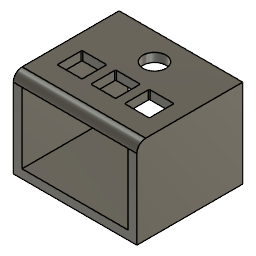
Lid (Autodesk Fusion 360 archive; units mm, degrees)
design "External1"
part number: 2026-05-08-13-42-59-027
Autodesk Fusion 360 part; units mm, degrees
other "DerivedContext1"
other "DerivedContext2"
sketch "sketch 238" plane through (0, 0, 0) normal (0, 1, 0) x (1, 0, 0)
  line L0 (35, -25) -> (-35, -25)
  line L1 (-35, -25) -> (-35, 25)
  line L2 (-35, 25) -> (35, 25)
  line L3 (35, 25) -> (35, -25)
  line L4 (35, -25) -> (-35, 25) construction
  line L5 (-35, -25) -> (35, 25) construction
extrude "Extrude1" add sketch "sketch 238" along normal blind 60
sketch "Sketch2" plane through (0, 0, 0) normal (0, -1, 0) x (1, 0, 0)
  line L0 (-35, -25) -> (35, -25)
  line L1 (35, -25) -> (35, 25)
  line L2 (35, 25) -> (-35, 25)
  line L3 (-35, 25) -> (-35, -25)
  line L4 (30, -20) -> (-30, -20)
  line L5 (-30, -20) -> (-30, 20)
  line L6 (-30, 20) -> (30, 20)
  line L7 (30, 20) -> (30, -20)
  line L8 (30, -20) -> (-30, 20) construction
  line L9 (-30, -20) -> (30, 20) construction
  dimension "d7" = 60
  dimension "d8" = 40
  constraint horizontal L4
  constraint perpendicular L4 L5
  constraint parallel L4 L6
  constraint parallel L5 L7
  constraint coincident L8 origin
  constraint coincident L9 origin
  measures "d7" distance of L5.end L6.end
  measures "d8" distance of L4.end L5.end
extrude "Extrude3" cut sketch "Sketch2" against normal blind 95 contours L4 L5 L6 L7
fillet "Fillet2" radius 5 1 edges at (0, 0, 25)
sketch "sketch 1124" plane through (28.575, 32.5, 25) normal (0, 0, 1) x (0, -1, 0)
  line L0 (3.025, -16.525) -> (16.025, -16.525)
  line L1 (2.525, -3.025) -> (2.525, -16.025)
  arc A0 (2.525, -16.025) -> (3.025, -16.525) centre (3.025, -16.025) ccw
  arc A1 (16.025, -16.525) -> (16.525, -16.025) centre (16.025, -16.025) ccw
  line L2 (3.025, -54.625) -> (16.025, -54.625)
  line L3 (0, 0) -> (19.05, 0)
  line L4 (16.525, -41.125) -> (16.525, -54.125)
  line L5 (2.525, -22.075) -> (2.525, -35.075)
  line L6 (0, -57.15) -> (0, 0)
  line L7 (16.525, -22.075) -> (16.525, -35.075)
  arc A2 (3.025, -2.525) -> (2.525, -3.025) centre (3.025, -3.025) ccw
  line L8 (3.025, -2.525) -> (16.025, -2.525)
  arc A3 (16.025, -54.625) -> (16.525, -54.125) centre (16.025, -54.125) ccw
  line L9 (3.025, -35.575) -> (16.025, -35.575)
  arc A4 (16.025, -35.575) -> (16.525, -35.075) centre (16.025, -35.075) ccw
  arc A5 (16.525, -41.125) -> (16.025, -40.625) centre (16.025, -41.125) ccw
  line L10 (19.05, -57.15) -> (19.05, 0)
  arc A6 (16.525, -3.025) -> (16.025, -2.525) centre (16.025, -3.025) ccw
  line L11 (16.525, -3.025) -> (16.525, -16.025)
  arc A7 (16.525, -22.075) -> (16.025, -21.575) centre (16.025, -22.075) ccw
  line L12 (0, -57.15) -> (19.05, -57.15)
  arc A8 (2.525, -35.075) -> (3.025, -35.575) centre (3.025, -35.075) ccw
  line L13 (3.025, -21.575) -> (16.025, -21.575)
  line L14 (2.525, -41.125) -> (2.525, -54.125)
  arc A9 (3.025, -40.625) -> (2.525, -41.125) centre (3.025, -41.125) ccw
  line L15 (3.025, -40.625) -> (16.025, -40.625)
  arc A10 (2.525, -54.125) -> (3.025, -54.625) centre (3.025, -54.125) ccw
  arc A11 (3.025, -21.575) -> (2.525, -22.075) centre (3.025, -22.075) ccw
extrude "Extrude4" cut sketch "sketch 1124" against normal blind 10 contours L0 L1 A0 A1 A2 L8 A6 L11 | L2 L4 A3 A5 L14 A9 L15 A10 | L5 L7 L9 A4 A7 A8 L13 A11
sketch "Sketch3" plane through (0, 0, 25) normal (0, 0, 1) x (-1, 0, 0)
  line L0 (25.55, -29.975) -> (12.55, -29.975)
  arc A0 (12.05, -29.475) -> (12.55, -29.975) centre (12.55, -29.475) ccw
  line L1 (12.05, -29.475) -> (12.05, -16.475)
  arc A1 (12.55, -15.975) -> (12.05, -16.475) centre (12.55, -16.475) ccw
  line L2 (12.55, -15.975) -> (25.55, -15.975)
  arc A2 (26.05, -16.475) -> (25.55, -15.975) centre (25.55, -16.475) ccw
  line L3 (26.05, -16.475) -> (26.05, -29.475)
  arc A3 (25.55, -29.975) -> (26.05, -29.475) centre (25.55, -29.475) ccw
  line L4 (-7, -29.475) -> (-7, -16.475)
  arc A4 (-6.5, -15.975) -> (-7, -16.475) centre (-6.5, -16.475) ccw
  line L5 (-6.5, -15.975) -> (6.5, -15.975)
  arc A5 (7, -16.475) -> (6.5, -15.975) centre (6.5, -16.475) ccw
  line L6 (7, -16.475) -> (7, -29.475)
  arc A6 (6.5, -29.975) -> (7, -29.475) centre (6.5, -29.475) ccw
  line L7 (6.5, -29.975) -> (-6.5, -29.975)
  arc A7 (-7, -29.475) -> (-6.5, -29.975) centre (-6.5, -29.475) ccw
  line L8 (-12.55, -29.975) -> (-25.55, -29.975)
  arc A8 (-26.05, -29.475) -> (-25.55, -29.975) centre (-25.55, -29.475) ccw
  line L9 (-26.05, -29.475) -> (-26.05, -16.475)
  arc A9 (-25.55, -15.975) -> (-26.05, -16.475) centre (-25.55, -16.475) ccw
  line L10 (-25.55, -15.975) -> (-12.55, -15.975)
  arc A10 (-12.05, -16.475) -> (-12.55, -15.975) centre (-12.55, -16.475) ccw
  line L11 (-12.05, -16.475) -> (-12.05, -29.475)
  arc A11 (-12.55, -29.975) -> (-12.05, -29.475) centre (-12.55, -29.475) ccw
  line L12 (35, -5) -> (-35, -5)
  line L13 (-35, -5) -> (-35, -60)
  line L14 (-35, -60) -> (35, -60)
  line L15 (35, -60) -> (35, -5)
  circle A12 centre (0, -45) radius 7.5
  dimension "d21" = 15
  measures "d21" diameter of A12
sketch "Sketch4" plane through (0, 0, 25) normal (0, 0, 1) x (-1, 0, 0)
  line L0 (25.55, -29.975) -> (12.55, -29.975)
  arc A0 (12.05, -29.475) -> (12.55, -29.975) centre (12.55, -29.475) ccw
  line L1 (12.05, -29.475) -> (12.05, -16.475)
  arc A1 (12.55, -15.975) -> (12.05, -16.475) centre (12.55, -16.475) ccw
  line L2 (12.55, -15.975) -> (25.55, -15.975)
  arc A2 (26.05, -16.475) -> (25.55, -15.975) centre (25.55, -16.475) ccw
  line L3 (26.05, -16.475) -> (26.05, -29.475)
  arc A3 (25.55, -29.975) -> (26.05, -29.475) centre (25.55, -29.475) ccw
  line L4 (-7, -29.475) -> (-7, -16.475)
  arc A4 (-6.5, -15.975) -> (-7, -16.475) centre (-6.5, -16.475) ccw
  line L5 (-6.5, -15.975) -> (6.5, -15.975)
  arc A5 (7, -16.475) -> (6.5, -15.975) centre (6.5, -16.475) ccw
  line L6 (7, -16.475) -> (7, -29.475)
  arc A6 (6.5, -29.975) -> (7, -29.475) centre (6.5, -29.475) ccw
  line L7 (6.5, -29.975) -> (-6.5, -29.975)
  arc A7 (-7, -29.475) -> (-6.5, -29.975) centre (-6.5, -29.475) ccw
  line L8 (-12.55, -29.975) -> (-25.55, -29.975)
  arc A8 (-26.05, -29.475) -> (-25.55, -29.975) centre (-25.55, -29.475) ccw
  line L9 (-26.05, -29.475) -> (-26.05, -16.475)
  arc A9 (-25.55, -15.975) -> (-26.05, -16.475) centre (-25.55, -16.475) ccw
  line L10 (-25.55, -15.975) -> (-12.55, -15.975)
  arc A10 (-12.05, -16.475) -> (-12.55, -15.975) centre (-12.55, -16.475) ccw
  line L11 (-12.05, -16.475) -> (-12.05, -29.475)
  arc A11 (-12.55, -29.975) -> (-12.05, -29.475) centre (-12.55, -29.475) ccw
  line L12 (35, -5) -> (-35, -5)
  line L13 (-35, -5) -> (-35, -60)
  line L14 (-35, -60) -> (35, -60)
  line L15 (35, -60) -> (35, -5)
  circle A12 centre (0, -45) radius 6.5
  dimension "d24" = 13
  measures "d24" diameter of A12
extrude "Extrude6" cut sketch "Sketch4" against normal blind 10 contours A12
